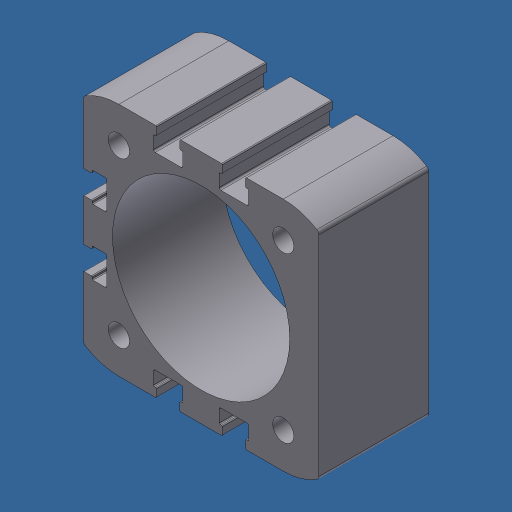
# Autodesk Inventor part: EXTRUSION,CYLINDER, ALUMINIUM, FESTO, 40MM
Saved by Autodesk Inventor 2024.3 (Build 283343000, 343)
## iProperties
Category: _
Manager: _
RuleStatus: InUse
Shininess: 64.0
Angle Display Precision: 2
Document Length Units: 11269
Document Angle Units: 11279
Document Time Units: 11290
Document Mass Units: 11286
Document Length Units Precision: 3
Document Angle Units Precision: 2
Part Number: EXTRUSION,CYLINDER, ALUMINIUM, FESTO, 40MM
Material: Aluminum, 6061-T6
Document SubType Name: Modeling
Created: 2019-07-31
Designer: -
Manufacturer: Standard
Standards Organization: Custom
Density: 2.71 g/cm^3
Mass: 92.4173 g
Surface Area: 148.046 cm^2
Volume: 34.1023 cm^3
Checked By: 00
Engr Approved By: _
User Status: Work In Process
Description: EXTRUSION, CYLINDER, ALUMINIUM, FESTO, 40MM
Mfg Approved By: -
Appearance: Aluminum (Flat)
BeforeDocSave0: Mass
BeforeDocSave1: PartFinishTrigger
Density: 0.0
Volumn: 0.0
Area: 0.0
PropertySet Name: Model Information
Control State: 0
Master: False
Checked Out: False
CN_MASS: 0.27
CN_SERVICEABLE: _
CL_runCount: 0
FIRST_DESCRIPTION: _
SECOND_DESCRIPTION: _
THIRD_DESCRIPTION: _
Author: -
Subject: _
Revision Number: A
Keywords: -
Autodesk Inventor part; units mm, degrees
ref_plane "YZ Plane" through (0, 0, 0) normal (1, 0, 0) x (0, 1, 0)
ref_plane "XZ Plane" through (0, 0, 0) normal (0, 1, 0) x (-1, 0, 0)
ref_plane "XY Plane" through (0, 0, 0) normal (0, 0, 1) x (1, 0, 0)
sketch "Sketch1" plane through (0, 0, 0) normal (0, 0, 1) x (1, 0, 0)
  arc A0 (4.2513, -12.4259) -> (12.0266, -10.2189) centre (4.2513, 2.3741) ccw
  line L0 (4.2513, -12.4259) -> (-4.2487, -12.4259)
  arc A1 (-4.4487, -12.2259) -> (-4.2487, -12.4259) centre (-4.2487, -12.2259) ccw
  line L1 (-4.4487, -12.2259) -> (-4.4487, -10.5759)
  arc A2 (-4.2487, -10.3759) -> (-4.4487, -10.5759) centre (-4.2487, -10.5759) ccw
  line L2 (-4.2487, -10.3759) -> (-3.9487, -10.3759)
  arc A3 (-3.9487, -10.3759) -> (-3.7487, -10.1759) centre (-3.9487, -10.1759) ccw
  line L3 (-3.7487, -10.1759) -> (-3.7487, -7.3759)
  arc A4 (-3.7487, -7.3759) -> (-4.1487, -6.9759) centre (-4.1487, -7.3759) ccw
  line L4 (-4.1487, -6.9759) -> (-10.1487, -6.9759)
  arc A5 (-10.1487, -6.9759) -> (-10.5487, -7.3759) centre (-10.1487, -7.3759) ccw
  line L5 (-10.5487, -7.3759) -> (-10.5487, -10.1759)
  arc A6 (-10.5487, -10.1759) -> (-10.3487, -10.3759) centre (-10.3487, -10.1759) ccw
  line L6 (-10.3487, -10.3759) -> (-10.0487, -10.3759)
  arc A7 (-9.8487, -10.5759) -> (-10.0487, -10.3759) centre (-10.0487, -10.5759) ccw
  line L7 (-9.8487, -10.5759) -> (-9.8487, -12.2259)
  arc A8 (-10.0487, -12.4259) -> (-9.8487, -12.2259) centre (-10.0487, -12.2259) ccw
  line L8 (-10.0487, -12.4259) -> (-19.4487, -12.4259)
  arc A9 (-19.6487, -12.2259) -> (-19.4487, -12.4259) centre (-19.4487, -12.2259) ccw
  line L9 (-19.6487, -12.2259) -> (-19.6487, -10.5759)
  arc A10 (-19.4487, -10.3759) -> (-19.6487, -10.5759) centre (-19.4487, -10.5759) ccw
  line L10 (-19.4487, -10.3759) -> (-19.1487, -10.3759)
  arc A11 (-19.1487, -10.3759) -> (-18.9487, -10.1759) centre (-19.1487, -10.1759) ccw
  line L11 (-18.9487, -10.1759) -> (-18.9487, -7.3759)
  arc A12 (-18.9487, -7.3759) -> (-19.3487, -6.9759) centre (-19.3487, -7.3759) ccw
  line L12 (-19.3487, -6.9759) -> (-25.3487, -6.9759)
  arc A13 (-25.3487, -6.9759) -> (-25.7487, -7.3759) centre (-25.3487, -7.3759) ccw
  line L13 (-25.7487, -7.3759) -> (-25.7487, -10.1759)
  arc A14 (-25.7487, -10.1759) -> (-25.5487, -10.3759) centre (-25.5487, -10.1759) ccw
  line L14 (-25.5487, -10.3759) -> (-25.2487, -10.3759)
  arc A15 (-25.0487, -10.5759) -> (-25.2487, -10.3759) centre (-25.2487, -10.5759) ccw
  line L15 (-25.0487, -10.5759) -> (-25.0487, -12.2259)
  arc A16 (-25.2487, -12.4259) -> (-25.0487, -12.2259) centre (-25.2487, -12.2259) ccw
  line L16 (-25.2487, -12.4259) -> (-33.7487, -12.4259)
  arc A17 (-41.5241, -10.2189) -> (-33.7487, -12.4259) centre (-33.7487, 2.3741) ccw
  arc A18 (-41.9987, -9.368) -> (-41.5241, -10.2189) centre (-40.9987, -9.368) ccw
  line L17 (-41.9987, -9.368) -> (-41.9987, 4.3241)
  arc A19 (-41.7987, 4.5241) -> (-41.9987, 4.3241) centre (-41.7987, 4.3241) ccw
  line L18 (-41.7987, 4.5241) -> (-40.1487, 4.5241)
  arc A20 (-39.9487, 4.3241) -> (-40.1487, 4.5241) centre (-40.1487, 4.3241) ccw
  line L19 (-39.9487, 4.3241) -> (-39.9487, 4.0241)
  arc A21 (-39.9487, 4.0241) -> (-39.7487, 3.8241) centre (-39.7487, 4.0241) ccw
  line L20 (-39.7487, 3.8241) -> (-36.9487, 3.8241)
  arc A22 (-36.9487, 3.8241) -> (-36.5487, 4.2241) centre (-36.9487, 4.2241) ccw
  line L21 (-36.5487, 4.2241) -> (-36.5487, 10.2241)
  arc A23 (-36.5487, 10.2241) -> (-36.9487, 10.6241) centre (-36.9487, 10.2241) ccw
  line L22 (-36.9487, 10.6241) -> (-39.7487, 10.6241)
  arc A24 (-39.7487, 10.6241) -> (-39.9487, 10.4241) centre (-39.7487, 10.4241) ccw
  line L23 (-39.9487, 10.4241) -> (-39.9487, 10.1241)
  arc A25 (-40.1487, 9.9241) -> (-39.9487, 10.1241) centre (-40.1487, 10.1241) ccw
  line L24 (-40.1487, 9.9241) -> (-41.7987, 9.9241)
  arc A26 (-41.9987, 10.1241) -> (-41.7987, 9.9241) centre (-41.7987, 10.1241) ccw
  line L25 (-41.9987, 10.1241) -> (-41.9987, 19.5241)
  arc A27 (-41.7987, 19.7241) -> (-41.9987, 19.5241) centre (-41.7987, 19.5241) ccw
  line L26 (-41.7987, 19.7241) -> (-40.1487, 19.7241)
  arc A28 (-39.9487, 19.5241) -> (-40.1487, 19.7241) centre (-40.1487, 19.5241) ccw
  line L27 (-39.9487, 19.5241) -> (-39.9487, 19.2241)
  arc A29 (-39.9487, 19.2241) -> (-39.7487, 19.0241) centre (-39.7487, 19.2241) ccw
  line L28 (-39.7487, 19.0241) -> (-36.9487, 19.0241)
  arc A30 (-36.9487, 19.0241) -> (-36.5487, 19.4241) centre (-36.9487, 19.4241) ccw
  line L29 (-36.5487, 19.4241) -> (-36.5487, 25.4241)
  arc A31 (-36.5487, 25.4241) -> (-36.9487, 25.8241) centre (-36.9487, 25.4241) ccw
  line L30 (-36.9487, 25.8241) -> (-39.7487, 25.8241)
  arc A32 (-39.7487, 25.8241) -> (-39.9487, 25.6241) centre (-39.7487, 25.6241) ccw
  line L31 (-39.9487, 25.6241) -> (-39.9487, 25.3241)
  arc A33 (-40.1487, 25.1241) -> (-39.9487, 25.3241) centre (-40.1487, 25.3241) ccw
  line L32 (-40.1487, 25.1241) -> (-41.7987, 25.1241)
  arc A34 (-41.9987, 25.3241) -> (-41.7987, 25.1241) centre (-41.7987, 25.3241) ccw
  line L33 (-41.9987, 25.3241) -> (-41.9987, 39.0162)
  arc A35 (-41.5241, 39.8671) -> (-41.9987, 39.0162) centre (-40.9987, 39.0162) ccw
  arc A36 (-33.7487, 42.0741) -> (-41.5241, 39.8671) centre (-33.7487, 27.2741) ccw
  line L34 (-33.7487, 42.0741) -> (-25.2487, 42.0741)
  arc A37 (-25.0487, 41.8741) -> (-25.2487, 42.0741) centre (-25.2487, 41.8741) ccw
  line L35 (-25.0487, 41.8741) -> (-25.0487, 40.2241)
  arc A38 (-25.2487, 40.0241) -> (-25.0487, 40.2241) centre (-25.2487, 40.2241) ccw
  line L36 (-25.2487, 40.0241) -> (-25.5487, 40.0241)
  arc A39 (-25.5487, 40.0241) -> (-25.7487, 39.8241) centre (-25.5487, 39.8241) ccw
  line L37 (-25.7487, 39.8241) -> (-25.7487, 37.0241)
  arc A40 (-25.7487, 37.0241) -> (-25.3487, 36.6241) centre (-25.3487, 37.0241) ccw
  line L38 (-25.3487, 36.6241) -> (-19.3487, 36.6241)
  arc A41 (-19.3487, 36.6241) -> (-18.9487, 37.0241) centre (-19.3487, 37.0241) ccw
  line L39 (-18.9487, 37.0241) -> (-18.9487, 39.8241)
  arc A42 (-18.9487, 39.8241) -> (-19.1487, 40.0241) centre (-19.1487, 39.8241) ccw
  line L40 (-19.1487, 40.0241) -> (-19.4487, 40.0241)
  arc A43 (-19.6487, 40.2241) -> (-19.4487, 40.0241) centre (-19.4487, 40.2241) ccw
  line L41 (-19.6487, 40.2241) -> (-19.6487, 41.8741)
  arc A44 (-19.4487, 42.0741) -> (-19.6487, 41.8741) centre (-19.4487, 41.8741) ccw
  line L42 (-19.4487, 42.0741) -> (-10.0487, 42.0741)
  arc A45 (-9.8487, 41.8741) -> (-10.0487, 42.0741) centre (-10.0487, 41.8741) ccw
  line L43 (-9.8487, 41.8741) -> (-9.8487, 40.2241)
  arc A46 (-10.0487, 40.0241) -> (-9.8487, 40.2241) centre (-10.0487, 40.2241) ccw
  line L44 (-10.0487, 40.0241) -> (-10.3487, 40.0241)
  arc A47 (-10.3487, 40.0241) -> (-10.5487, 39.8241) centre (-10.3487, 39.8241) ccw
  line L45 (-10.5487, 39.8241) -> (-10.5487, 37.0241)
  arc A48 (-10.5487, 37.0241) -> (-10.1487, 36.6241) centre (-10.1487, 37.0241) ccw
  line L46 (-10.1487, 36.6241) -> (-4.1487, 36.6241)
  arc A49 (-4.1487, 36.6241) -> (-3.7487, 37.0241) centre (-4.1487, 37.0241) ccw
  line L47 (-3.7487, 37.0241) -> (-3.7487, 39.8241)
  arc A50 (-3.7487, 39.8241) -> (-3.9487, 40.0241) centre (-3.9487, 39.8241) ccw
  line L48 (-3.9487, 40.0241) -> (-4.2487, 40.0241)
  arc A51 (-4.4487, 40.2241) -> (-4.2487, 40.0241) centre (-4.2487, 40.2241) ccw
  line L49 (-4.4487, 40.2241) -> (-4.4487, 41.8741)
  arc A52 (-4.2487, 42.0741) -> (-4.4487, 41.8741) centre (-4.2487, 41.8741) ccw
  line L50 (-4.2487, 42.0741) -> (4.2513, 42.0741)
  arc A53 (4.2513, 36.2826) -> (4.2513, 31.3656) centre (4.2513, 33.8241) ccw
  arc A54 (4.2513, 31.3656) -> (4.2513, 36.2826) centre (4.2513, 33.8241) ccw
  arc A55 (-33.7487, 36.2826) -> (-33.7487, 31.3656) centre (-33.7487, 33.8241) ccw
  arc A56 (-33.7487, 31.3656) -> (-33.7487, 36.2826) centre (-33.7487, 33.8241) ccw
  arc A57 (-33.7487, -1.7174) -> (-33.7487, -6.6344) centre (-33.7487, -4.1759) ccw
  arc A58 (-33.7487, -6.6344) -> (-33.7487, -1.7174) centre (-33.7487, -4.1759) ccw
  arc A59 (4.2513, -6.6344) -> (4.2513, -1.7174) centre (4.2513, -4.1759) ccw
  arc A60 (4.2513, -1.7174) -> (4.2513, -6.6344) centre (4.2513, -4.1759) ccw
  arc A61 (12.0266, -10.2189) -> (12.5013, -9.368) centre (11.5013, -9.368) ccw
  arc A62 (-41.7987, 4.5241) -> (-41.9987, 4.3241) centre (-41.7987, 4.3241) ccw
  line L51 (-41.9987, -9.368) -> (-41.9987, 4.3241)
  arc A63 (-41.9987, -9.368) -> (-41.5241, -10.2189) centre (-40.9987, -9.368) ccw
  arc A64 (-41.5241, -10.2189) -> (-33.7487, -12.4259) centre (-33.7487, 2.3741) ccw
  line L52 (-25.2487, -12.4259) -> (-33.7487, -12.4259)
  arc A65 (-25.2487, -12.4259) -> (-25.0487, -12.2259) centre (-25.2487, -12.2259) ccw
  line L53 (-25.0487, -10.5759) -> (-25.0487, -12.2259)
  arc A66 (-25.0487, -10.5759) -> (-25.2487, -10.3759) centre (-25.2487, -10.5759) ccw
  line L54 (-25.5487, -10.3759) -> (-25.2487, -10.3759)
  arc A67 (-25.7487, -10.1759) -> (-25.5487, -10.3759) centre (-25.5487, -10.1759) ccw
  line L55 (-25.7487, -7.3759) -> (-25.7487, -10.1759)
  arc A68 (-25.3487, -6.9759) -> (-25.7487, -7.3759) centre (-25.3487, -7.3759) ccw
  line L56 (-19.3487, -6.9759) -> (-25.3487, -6.9759)
  arc A69 (-18.9487, -7.3759) -> (-19.3487, -6.9759) centre (-19.3487, -7.3759) ccw
  line L57 (-18.9487, -10.1759) -> (-18.9487, -7.3759)
  arc A70 (-19.1487, -10.3759) -> (-18.9487, -10.1759) centre (-19.1487, -10.1759) ccw
  line L58 (-19.4487, -10.3759) -> (-19.1487, -10.3759)
  arc A71 (-19.4487, -10.3759) -> (-19.6487, -10.5759) centre (-19.4487, -10.5759) ccw
  line L59 (-19.6487, -12.2259) -> (-19.6487, -10.5759)
  arc A72 (-19.6487, -12.2259) -> (-19.4487, -12.4259) centre (-19.4487, -12.2259) ccw
  line L60 (-10.0487, -12.4259) -> (-19.4487, -12.4259)
  arc A73 (-10.0487, -12.4259) -> (-9.8487, -12.2259) centre (-10.0487, -12.2259) ccw
  line L61 (-9.8487, -10.5759) -> (-9.8487, -12.2259)
  arc A74 (-9.8487, -10.5759) -> (-10.0487, -10.3759) centre (-10.0487, -10.5759) ccw
  line L62 (-10.3487, -10.3759) -> (-10.0487, -10.3759)
  arc A75 (-10.5487, -10.1759) -> (-10.3487, -10.3759) centre (-10.3487, -10.1759) ccw
  line L63 (-10.5487, -7.3759) -> (-10.5487, -10.1759)
  arc A76 (-10.1487, -6.9759) -> (-10.5487, -7.3759) centre (-10.1487, -7.3759) ccw
  line L64 (-4.1487, -6.9759) -> (-10.1487, -6.9759)
  arc A77 (-3.7487, -7.3759) -> (-4.1487, -6.9759) centre (-4.1487, -7.3759) ccw
  line L65 (-3.7487, -10.1759) -> (-3.7487, -7.3759)
  arc A78 (-3.9487, -10.3759) -> (-3.7487, -10.1759) centre (-3.9487, -10.1759) ccw
  line L66 (-4.2487, -10.3759) -> (-3.9487, -10.3759)
  arc A79 (-4.2487, -10.3759) -> (-4.4487, -10.5759) centre (-4.2487, -10.5759) ccw
  line L67 (-4.4487, -12.2259) -> (-4.4487, -10.5759)
  arc A80 (-4.4487, -12.2259) -> (-4.2487, -12.4259) centre (-4.2487, -12.2259) ccw
  line L68 (4.2513, -12.4259) -> (-4.2487, -12.4259)
  arc A81 (4.2513, -12.4259) -> (12.0266, -10.2189) centre (4.2513, 2.3741) ccw
  arc A82 (12.0266, -10.2189) -> (12.5013, -9.368) centre (11.5013, -9.368) ccw
  line L69 (12.5013, 39.0162) -> (12.5013, -9.368)
  arc A83 (12.5013, 39.0162) -> (12.0266, 39.8671) centre (11.5013, 39.0162) ccw
  arc A84 (12.0266, 39.8671) -> (4.2513, 42.0741) centre (4.2513, 27.2741) ccw
  line L70 (-4.2487, 42.0741) -> (4.2513, 42.0741)
  arc A85 (-4.2487, 42.0741) -> (-4.4487, 41.8741) centre (-4.2487, 41.8741) ccw
  line L71 (-4.4487, 40.2241) -> (-4.4487, 41.8741)
  arc A86 (-4.4487, 40.2241) -> (-4.2487, 40.0241) centre (-4.2487, 40.2241) ccw
  line L72 (-3.9487, 40.0241) -> (-4.2487, 40.0241)
  arc A87 (-3.7487, 39.8241) -> (-3.9487, 40.0241) centre (-3.9487, 39.8241) ccw
  line L73 (-3.7487, 37.0241) -> (-3.7487, 39.8241)
  arc A88 (-4.1487, 36.6241) -> (-3.7487, 37.0241) centre (-4.1487, 37.0241) ccw
  line L74 (-10.1487, 36.6241) -> (-4.1487, 36.6241)
  arc A89 (-10.5487, 37.0241) -> (-10.1487, 36.6241) centre (-10.1487, 37.0241) ccw
  line L75 (-10.5487, 39.8241) -> (-10.5487, 37.0241)
  arc A90 (-10.3487, 40.0241) -> (-10.5487, 39.8241) centre (-10.3487, 39.8241) ccw
  line L76 (-10.0487, 40.0241) -> (-10.3487, 40.0241)
  arc A91 (-10.0487, 40.0241) -> (-9.8487, 40.2241) centre (-10.0487, 40.2241) ccw
  line L77 (-9.8487, 41.8741) -> (-9.8487, 40.2241)
  arc A92 (-9.8487, 41.8741) -> (-10.0487, 42.0741) centre (-10.0487, 41.8741) ccw
  line L78 (-19.4487, 42.0741) -> (-10.0487, 42.0741)
  arc A93 (-19.4487, 42.0741) -> (-19.6487, 41.8741) centre (-19.4487, 41.8741) ccw
  line L79 (-19.6487, 40.2241) -> (-19.6487, 41.8741)
  arc A94 (-19.6487, 40.2241) -> (-19.4487, 40.0241) centre (-19.4487, 40.2241) ccw
  line L80 (-19.1487, 40.0241) -> (-19.4487, 40.0241)
  arc A95 (-18.9487, 39.8241) -> (-19.1487, 40.0241) centre (-19.1487, 39.8241) ccw
  line L81 (-18.9487, 37.0241) -> (-18.9487, 39.8241)
  arc A96 (-19.3487, 36.6241) -> (-18.9487, 37.0241) centre (-19.3487, 37.0241) ccw
  line L82 (-25.3487, 36.6241) -> (-19.3487, 36.6241)
  arc A97 (-25.7487, 37.0241) -> (-25.3487, 36.6241) centre (-25.3487, 37.0241) ccw
  line L83 (-25.7487, 39.8241) -> (-25.7487, 37.0241)
  arc A98 (-25.5487, 40.0241) -> (-25.7487, 39.8241) centre (-25.5487, 39.8241) ccw
  line L84 (-25.2487, 40.0241) -> (-25.5487, 40.0241)
  arc A99 (-25.2487, 40.0241) -> (-25.0487, 40.2241) centre (-25.2487, 40.2241) ccw
  line L85 (-25.0487, 41.8741) -> (-25.0487, 40.2241)
  arc A100 (-25.0487, 41.8741) -> (-25.2487, 42.0741) centre (-25.2487, 41.8741) ccw
  line L86 (-33.7487, 42.0741) -> (-25.2487, 42.0741)
  arc A101 (-33.7487, 42.0741) -> (-41.5241, 39.8671) centre (-33.7487, 27.2741) ccw
  arc A102 (-41.5241, 39.8671) -> (-41.9987, 39.0162) centre (-40.9987, 39.0162) ccw
  line L87 (-41.9987, 25.3241) -> (-41.9987, 39.0162)
  arc A103 (-41.9987, 25.3241) -> (-41.7987, 25.1241) centre (-41.7987, 25.3241) ccw
  line L88 (-40.1487, 25.1241) -> (-41.7987, 25.1241)
  arc A104 (-40.1487, 25.1241) -> (-39.9487, 25.3241) centre (-40.1487, 25.3241) ccw
  line L89 (-39.9487, 25.6241) -> (-39.9487, 25.3241)
  arc A105 (-39.7487, 25.8241) -> (-39.9487, 25.6241) centre (-39.7487, 25.6241) ccw
  line L90 (-36.9487, 25.8241) -> (-39.7487, 25.8241)
  arc A106 (-36.5487, 25.4241) -> (-36.9487, 25.8241) centre (-36.9487, 25.4241) ccw
  line L91 (-36.5487, 19.4241) -> (-36.5487, 25.4241)
  arc A107 (-36.9487, 19.0241) -> (-36.5487, 19.4241) centre (-36.9487, 19.4241) ccw
  line L92 (-39.7487, 19.0241) -> (-36.9487, 19.0241)
  arc A108 (-39.9487, 19.2241) -> (-39.7487, 19.0241) centre (-39.7487, 19.2241) ccw
  line L93 (-39.9487, 19.5241) -> (-39.9487, 19.2241)
  arc A109 (-39.9487, 19.5241) -> (-40.1487, 19.7241) centre (-40.1487, 19.5241) ccw
  line L94 (-41.7987, 19.7241) -> (-40.1487, 19.7241)
  arc A110 (-41.7987, 19.7241) -> (-41.9987, 19.5241) centre (-41.7987, 19.5241) ccw
  line L95 (-41.9987, 10.1241) -> (-41.9987, 19.5241)
  arc A111 (-41.9987, 10.1241) -> (-41.7987, 9.9241) centre (-41.7987, 10.1241) ccw
  line L96 (-40.1487, 9.9241) -> (-41.7987, 9.9241)
  arc A112 (-40.1487, 9.9241) -> (-39.9487, 10.1241) centre (-40.1487, 10.1241) ccw
  line L97 (-39.9487, 10.4241) -> (-39.9487, 10.1241)
  arc A113 (-39.7487, 10.6241) -> (-39.9487, 10.4241) centre (-39.7487, 10.4241) ccw
  line L98 (-36.9487, 10.6241) -> (-39.7487, 10.6241)
  arc A114 (-36.5487, 10.2241) -> (-36.9487, 10.6241) centre (-36.9487, 10.2241) ccw
  line L99 (-36.5487, 4.2241) -> (-36.5487, 10.2241)
  arc A115 (-36.9487, 3.8241) -> (-36.5487, 4.2241) centre (-36.9487, 4.2241) ccw
  line L100 (-39.7487, 3.8241) -> (-36.9487, 3.8241)
  arc A116 (-39.9487, 4.0241) -> (-39.7487, 3.8241) centre (-39.7487, 4.0241) ccw
  line L101 (-39.9487, 4.3241) -> (-39.9487, 4.0241)
  arc A117 (-39.9487, 4.3241) -> (-40.1487, 4.5241) centre (-40.1487, 4.3241) ccw
  line L102 (-41.7987, 4.5241) -> (-40.1487, 4.5241)
  circle A118 centre (-14.7487, 14.8241) radius 20.5
  point P0 (0.0013, 42.0741)
  point P1 (8.2925, 41.5117)
  dimension "d1" = 41
  constraints: 4 coincident, 1 centre point, 1 midpoint, 1 point on circle, 3 other
  measures "d1" diameter of A118
extrude "FESTO, 40MM" add sketch "Sketch1" along normal blind 25.4 contours L0 A1 L1 A2 L2 A3 L3 A4 L4 A5 L5 A6 L6 A7 L7 A8 L8 A9 L9 A10 L10 A11 L11 A12 L12 A13 L13 A14 L14 A15 L15 A16 L16 A17 A18 L17 A19 L18 A20 L19 A21 L20 A22 L21 A23 L22 A24 L23 A25 L24 A26 L25 A27 L26 A28 L27 A29 L28 A30 L29 A31 L30 A32 L31 A33 L32 A34 L33 A35 A36 L34 A37 L35 A38 L36 A39 L37 A40 L38 A41 L39 A42 L40 A43 L41 A44 L42 A45 L43 A46 L44 A47 L45 A48 L46 A49 L47 A50 L48 A51 L49 A52 L50 A84 A83 L69 A61 A0 | A54 A53 | A56 A55 | A58 A57 | A60 A59
hole "Hole1" at (4.2513, 33.8241, 0) at (-33.7487, 33.8241, 0) at (-33.7487, -4.1759, 0) at (4.2513, -4.1759, 0) direction (0, 0, 1) diameter 4.91 end through all
